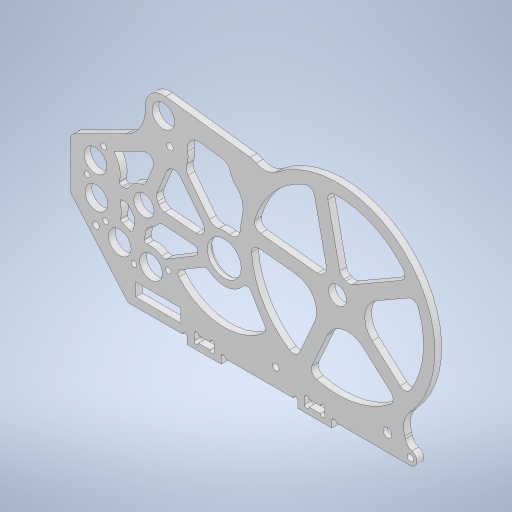
# Autodesk Inventor part: 右フレーム
Saved by Autodesk Inventor 2023.1 (Build 271208000, 208)
## iProperties
Created: 2022-06-19
Part Number: 右フレーム
Material: アルミニウム 2014-T6
Document SubType Name: Modeling
Designer: muzho
Density: 2.78927 g/cm^3
Appearance: サテン
Mass: 58.0664 g
Surface Area: 187.027 cm^2
Volume: 20.8178 cm^3
Author: muzho
Autodesk Inventor part; units mm, degrees
ref_plane "YZ Plane" through (0, 0, 0) normal (1, 0, 0) x (0, 1, 0)
ref_plane "XZ Plane" through (0, 0, 0) normal (0, 1, 0) x (-1, 0, 0)
ref_plane "XY Plane" through (0, 0, 0) normal (0, 0, 1) x (1, 0, 0)
sketch "スケッチ1" plane through (0, 0, 0) normal (0, 0, 1) x (1, 0, 0)
  circle A0 centre (-51.0684, 48.1873) radius 1.3
  circle A1 centre (-58.3027, 33.9162) radius 1.3
  circle A2 centre (-50.1964, 20.1218) radius 1.3
  circle A3 centre (-37.7457, 10.0728) radius 1.3
  circle A4 centre (-22.565, 15.1272) radius 1.3
  circle A5 centre (-33.2954, 34.6933) radius 22.3153 construction
  circle A6 centre (2.1359, 32) radius 30.9835 construction
  circle A7 centre (52, 42.9528) radius 41.9528 construction
  circle A8 centre (2.1208, 32.0012) radius 10.5
  circle A9 centre (-33.2954, 34.6933) radius 6.4335 construction
  circle A10 centre (-54.6856, 41.0518) radius 5.025
  circle A11 centre (-54.2496, 27.019) radius 5.025
  circle A12 centre (-43.9711, 15.0973) radius 5.025
  circle A13 centre (-30.1554, 12.6) radius 5.025
  circle A14 centre (-21.8214, 62.7533) radius 3
  circle A15 centre (-21.8214, 62.7533) radius 8
  line L0 (-21.8214, 62.7533) -> (-51.0684, 48.1873) construction
  line L1 (-33.3165, 55.1292) -> (-46.2281, 48.6988)
  arc A16 (-46.2281, 48.6988) -> (-46.7797, 47.8761) centre (-45.7823, 47.8037) ccw
  arc A17 (-52.9854, 52.0364) -> (-52.4722, 52.2518) centre (-51.0684, 48.1873) ccw construction
  arc A18 (-45.8061, 47.5867) -> (-65.5671, 39.279) centre (-54.6856, 41.0518) ccw construction
  line L2 (-65.7532, 43.7746) -> (-65.4452, 23.4769)
  arc A19 (-63.3575, 39.1831) -> (-63.6558, 28.9529) centre (-58.3027, 33.9162) ccw construction
  arc A20 (-45.2817, 33.4322) -> (-57.345, 16.4375) centre (-54.2496, 27.019) ccw construction
  arc A21 (-54.981, 15.674) -> (-41.5533, 4.3407) centre (-43.9711, 15.0973) ccw construction
  arc A22 (-65.4452, 23.4769) -> (-65.2027, 22.8391) centre (-64.4453, 23.4921) ccw
  line L3 (-65.2027, 22.8391) -> (-40.6377, -5.653)
  arc A23 (-40.6377, -5.653) -> (-39.8804, -6) centre (-39.8804, -5) ccw
  line L4 (-39.8804, -6) -> (84.0728, -6)
  line L5 (-6.7219, 36.0268) -> (-6.7219, -6.1434) construction
  line L6 (-37.0636, -3) -> (111.1776, -3) construction
  circle A24 centre (-10.2219, -3) radius 1
  circle A25 centre (-10.2219, -6) radius 1
  circle A26 centre (-15.2219, -6) radius 1
  line L7 (-11.2219, -3) -> (-11.2219, -6)
  circle A27 centre (-3.2219, -3) radius 1
  line L8 (-2.2219, -3) -> (-2.2219, -6)
  circle A28 centre (-3.2219, -6) radius 1
  circle A29 centre (1.7781, -6) radius 1
  line L9 (-9.2219, -3) -> (-4.2219, -3)
  line L10 (-14.2219, -6) -> (-14.2219, -9)
  line L11 (-14.2219, -9) -> (-7.7219, -9)
  line L12 (0.7781, -9) -> (-7.7219, -9)
  line L13 (0.7781, -6) -> (0.7781, -9)
  circle A30 centre (-33.2954, 34.6933) radius 4.5
  circle A31 centre (-33.2954, 34.6933) radius 7.5
  line L14 (-54.6856, 41.0518) -> (-54.2496, 27.019) construction
  line L15 (-54.4676, 34.0354) -> (-33.2954, 34.6933) construction
  arc A32 (-46.934, 49.3692) -> (-46.3247, 48.2383) centre (-44.0496, 50.1938) ccw
  arc A33 (-44.0483, 38.1537) -> (-46.3247, 48.2383) centre (-54.6856, 41.0518) ccw
  line L16 (-43.0524, 36.8913) -> (-42.313, 36.9143)
  line L17 (-42.8971, 31.8937) -> (-42.1577, 31.9167)
  arc A34 (-44.0483, 38.1537) -> (-43.0524, 36.8913) centre (-43.0835, 37.8908) ccw
  arc A35 (-42.8971, 31.8937) -> (-43.8127, 30.5719) centre (-42.8661, 30.8942) ccw
  arc A36 (-43.5733, 24.2678) -> (-43.8127, 30.5719) centre (-54.2496, 27.019) ccw
  arc A37 (-43.5733, 24.2678) -> (-42.7563, 23.0298) centre (-42.605, 24.0183) ccw
  arc A38 (-39.5768, 21.8123) -> (-42.7563, 23.0298) centre (-43.9711, 15.0973) ccw
  arc A39 (-42.313, 36.9143) -> (-39.8031, 38.4215) centre (-42.4062, 39.9128) ccw
  arc A40 (-39.5591, 30.5682) -> (-42.1577, 31.9167) centre (-42.0645, 28.9181) ccw
  arc A41 (-39.5768, 21.8123) -> (-38.0451, 22.4712) centre (-39.0292, 22.649) ccw
  line L18 (-38.0451, 22.4712) -> (-37.3465, 26.3363)
  line L19 (-43.9711, 15.0973) -> (-30.1554, 12.6) construction
  line L20 (-37.0632, 13.8486) -> (-33.2954, 34.6933) construction
  line L21 (-32.4262, 25.4469) -> (-33.1249, 21.5818)
  arc A42 (-33.1249, 21.5818) -> (-31.9208, 20.4284) centre (-32.1408, 21.4039) ccw
  arc A43 (-25.4982, 19.1354) -> (-31.9208, 20.4284) centre (-30.1554, 12.6) ccw
  arc A44 (-37.3465, 26.3363) -> (-38.2977, 29.1052) centre (-40.2986, 26.8699) ccw
  arc A45 (-30.5659, 27.7076) -> (-32.4262, 25.4469) centre (-29.4741, 24.9133) ccw
  arc A46 (-32.898, 62.0405) -> (-29.1429, 65.9774) centre (-36.4645, 69.2016) ccw
  line L22 (-21.8214, 62.7533) -> (-33.2954, 34.6933) construction
  line L23 (-29.2023, 51.3083) -> (-32.2241, 43.9183)
  line L24 (-23.2251, 52.7152) -> (-27.5961, 42.0259)
  arc A47 (-34.5136, 42.0937) -> (-32.2241, 43.9183) centre (-35.0009, 45.0538) ccw
  arc A48 (-27.5961, 42.0259) -> (-27.241, 39.1198) centre (-24.8193, 40.8904) ccw
  arc A49 (-29.2023, 51.3083) -> (-33.3165, 55.1292) centre (-31.9791, 52.4438) ccw
  circle A50 centre (2.1208, 32.0012) radius 7.5
  circle A51 centre (2.1208, 32.0012) radius 8.5
  arc A52 (-25.4982, 19.1354) -> (-23.3071, 19.05) centre (-24.3375, 20.7641) ccw
  line L25 (-23.3071, 19.05) -> (-10.4064, 26.8046)
  line L26 (-30.1554, 12.6) -> (2.1208, 32.0012) construction
  arc A53 (-26.6272, 38.1263) -> (-24.1874, 36.5081) centre (-23.96, 39.4995) ccw
  arc A54 (-24.5663, 31.5225) -> (-27.2228, 30.2917) centre (-24.7937, 28.5311) ccw
  line L27 (-24.1874, 36.5081) -> (-10.2124, 35.4459)
  line L28 (-24.5663, 31.5225) -> (-11.2852, 30.513)
  line L29 (-33.2954, 34.6933) -> (2.1208, 32.0012) construction
  arc A55 (-10.4064, 26.8046) -> (-11.2852, 30.513) centre (-11.4368, 28.5187) ccw
  circle A56 centre (-54.6856, 41.0518) radius 14 construction
  line L30 (42, 44.1233) -> (42, -23.5713) construction
  circle A57 centre (38.5, -3) radius 1
  circle A58 centre (38.5, -6) radius 1
  circle A59 centre (33.5, -6) radius 1
  line L31 (37.5, -3) -> (37.5, -6)
  line L32 (34.5, -6) -> (34.5, -9)
  line L33 (34.5, -9) -> (42, -9)
  circle A60 centre (45.5, -3) radius 1
  line L34 (46.5, -3) -> (46.5, -6)
  circle A61 centre (45.5, -6) radius 1
  line L35 (49.5, -6) -> (49.5, -9)
  line L36 (49.5, -9) -> (42, -9)
  circle A62 centre (50.5, -6) radius 1
  line L37 (39.5, -3) -> (44.5, -3)
  circle A63 centre (52, 42.9528) radius 4.025
  circle A64 centre (52, 42.9528) radius 8.025
  arc A65 (83.7206, 13.9916) -> (24.9838, 76.3454) centre (52, 42.9528) ccw
  line L38 (52, 42.9528) -> (49.2725, 42.9528) construction
  arc A66 (55.6469, 50.1013) -> (58.5102, 50.1755) centre (57.0102, 52.7736) ccw
  line L39 (58.5102, 50.1755) -> (80.3207, 62.7679)
  arc A67 (80.3207, 62.7679) -> (81.1227, 67.2896) centre (78.8207, 65.3659) ccw
  arc A68 (61.5102, 44.9794) -> (60.0142, 42.5368) centre (63.0102, 42.3813) ccw
  arc A69 (87.6377, 56.0054) -> (83.3207, 57.5717) centre (84.8207, 54.9736) ccw
  line L40 (61.5102, 44.9794) -> (83.3207, 57.5717)
  line L41 (52, 42.9528) -> (85.5729, 62.3361) construction
  line L42 (52, 42.9528) -> (90.7666, 42.9528) construction
  line L43 (47.1425, 51.3763) -> (41.9063, 76.0106)
  arc A70 (46.3283, 48.6302) -> (47.1425, 51.3763) centre (44.2081, 50.7526) ccw
  arc A71 (41.9063, 76.0106) -> (37.8537, 78.1706) centre (38.9719, 75.3868) ccw
  arc A72 (50.5989, 80.8797) -> (47.7752, 77.258) centre (50.7097, 77.8818) ccw
  line L44 (53.0114, 52.6238) -> (47.7752, 77.258)
  arc A73 (53.0114, 52.6238) -> (54.8721, 50.4462) centre (55.9458, 53.2475) ccw
  line L45 (42.4877, 40.936) -> (17.4411, 43.5686)
  arc A74 (44.8478, 39.3131) -> (42.4877, 40.936) centre (42.1741, 37.9525) ccw
  arc A75 (17.4411, 43.5686) -> (14.1344, 40.3818) centre (17.1275, 40.585) ccw
  arc A76 (15.4964, 53.3403) -> (18.0683, 49.5357) centre (18.3818, 52.5193) ccw
  line L46 (43.1149, 46.9032) -> (18.0683, 49.5357)
  arc A77 (43.1149, 46.9032) -> (45.7609, 48) centre (43.4285, 49.8867) ccw
  line L47 (50.9786, 33.2829) -> (40.7351, 10.2756)
  arc A78 (53.2514, 35.026) -> (50.9786, 33.2829) centre (53.7192, 32.0627) ccw
  arc A79 (40.7351, 10.2756) -> (42.7441, 6.146) centre (43.4757, 9.0554) ccw
  arc A80 (30.8406, 11.4457) -> (35.2538, 12.716) centre (32.5132, 13.9362) ccw
  line L48 (45.4973, 35.7233) -> (35.2538, 12.716)
  arc A81 (45.4973, 35.7233) -> (45.2719, 38.5787) centre (42.7567, 36.9435) ccw
  line L49 (60.881, 38.9932) -> (79.5968, 22.1414)
  arc A82 (59.9256, 41.6934) -> (60.881, 38.9932) centre (62.8884, 41.2226) ccw
  arc A83 (79.5968, 22.1414) -> (84.1451, 22.776) centre (81.6042, 24.3708) ccw
  arc A84 (75.4264, 13.0928) -> (75.582, 17.6825) centre (73.5746, 15.4531) ccw
  line L50 (56.8662, 34.5343) -> (75.582, 17.6825)
  arc A85 (56.8662, 34.5343) -> (54.0809, 35.2023) centre (54.8588, 32.3049) ccw
  circle A86 centre (52, 42.9528) radius 37.9528
  circle A87 centre (-33.5773, 1) radius 1.5 construction
  circle A88 centre (-33.5773, 1) radius 3 construction
  line L51 (-39.8804, -5) -> (-33.5773, 1) construction
  circle A89 centre (24.8719, 2) radius 1.5
  circle A90 centre (24.8719, 2) radius 3
  line L52 (24.8719, 10.9511) -> (24.8719, -6.9511) construction
  circle A91 centre (84.0728, -3) radius 1.5
  circle A92 centre (84.0728, -3) radius 3
  arc A93 (-17.1874, 53.5456) -> (-23.2251, 52.7152) centre (-19.9659, 51.3824) ccw
  line L53 (-21.8214, 62.7533) -> (2.1208, 32.0012) construction
  line L54 (-17.1874, 53.5456) -> (-7.3085, 40.8568)
  arc A94 (-10.2124, 35.4459) -> (-7.3085, 40.8568) centre (-9.9579, 38.794) ccw
  arc A95 (10.184, 52.7694) -> (9.1488, 45.9046) centre (52, 42.9528) ccw
  arc A96 (-4.6743, 23.9963) -> (10.5141, 25.6922) centre (2.1208, 32.0012) ccw
  arc A97 (-4.6743, 23.9963) -> (-6.999, 24.1858) centre (-5.9686, 22.4716) ccw
  line L55 (-6.999, 24.1858) -> (-17.3917, 17.9387)
  arc A98 (-17.3917, 17.9387) -> (-17.8825, 14.9261) centre (-16.3614, 16.2245) ccw
  arc A99 (-20.5941, 11.3055) -> (-18.526, 16.6024) centre (-22.565, 15.1272) ccw construction
  arc A100 (-17.8825, 14.9261) -> (19.7697, 12.5022) centre (2.1208, 32.0012) ccw
  arc A101 (13.8269, 25.5208) -> (10.5141, 25.6922) centre (12.1128, 24.4905) ccw
  line L56 (13.8269, 25.5208) -> (20.1417, 15.0154)
  arc A102 (19.7697, 12.5022) -> (20.1417, 15.0154) centre (18.4276, 13.985) ccw
  arc A103 (16.2511, 75.4723) -> (24.9838, 76.3454) centre (19.952, 82.5648) ccw
  circle A104 centre (12.5499, 68.38) radius 4
  circle A105 centre (12.5499, 68.38) radius 8
  circle A106 centre (74.0428, 1.5165) radius 2
  arc A107 (76.7818, -6) -> (71.3037, -6) centre (74.0428, 1.5165) ccw
  arc A108 (83.7206, 13.9916) -> (81.6262, 4.0643) centre (91.1055, 7.2491) ccw
  arc A109 (81.8996, 3.0231) -> (84.8251, -0.0958) centre (85.8281, 3.7764) ccw
  arc A110 (-64.0909, 46.5055) -> (-65.7532, 43.7746) centre (-62.7535, 43.8201) ccw
  line L57 (-64.0909, 46.5055) -> (-32.898, 62.0405)
  circle A111 centre (2.1208, 32.0012) radius 11.5 construction
  circle A112 centre (74.0428, 1.5165) radius 3
  circle A113 centre (74.0428, 1.5165) radius 4
  circle A114 centre (12.5499, 68.38) radius 2
  circle A115 centre (-21.8214, 62.7533) radius 1.5
  circle A116 centre (-54.4309, 16.4709) radius 1.5
  circle A117 centre (-54.4309, 16.4709) radius 3
  arc A118 (-58.2926, 17.5135) -> (-53.5618, 12.5665) centre (-54.4309, 16.4709) ccw construction
  line L58 (-54.2496, 27.019) -> (-43.9711, 15.0973)
  line L59 (-54.4309, 16.4709) -> (-49.1103, 21.0581)
  arc A119 (68.9958, 49.3012) -> (67.3045, 33.2095) centre (73.9958, 40.6409) ccw
  arc A120 (63.2897, 28.7506) -> (47.4629, 25.3865) centre (56.5984, 21.3192) ccw
  arc A121 (41.9816, 27.827) -> (33.8915, 41.8396) centre (32.8462, 31.8943) ccw
  circle A122 centre (-24.7192, 72.9643) radius 4 construction
  arc A123 (-27.2542, 68.6256) -> (-20.283, 70.6039) centre (-24.7192, 72.9643) ccw
  arc A124 (-29.0291, 66.2245) -> (-17.5115, 69.493) centre (-24.7192, 72.9643) ccw construction
  arc A125 (-17.5115, 69.493) -> (-29.0291, 66.2245) centre (-24.7192, 72.9643) ccw
  arc A126 (-40.9817, 58.0146) -> (-32.7016, 72.4347) centre (-47.6687, 71.4416) ccw
  line L60 (-23.7425, 80.9044) -> (13.5266, 76.3201)
  arc A127 (4.7383, 66.6541) -> (1.3208, 69.7612) centre (0.8325, 65.7911) ccw
  line L61 (1.3208, 69.7612) -> (-8.6288, 70.9851)
  arc A128 (-8.6288, 70.9851) -> (-14.0785, 64.7651) centre (-9.2392, 66.0225) ccw
  arc A129 (10.184, 52.7694) -> (7.1716, 62.4577) centre (0.4487, 55.0548) ccw
  arc A130 (4.3203, 42.2682) -> (9.1488, 45.9046) centre (5.1582, 46.1794) ccw
  arc A131 (-14.409, 59.7438) -> (-13.8591, 55.7818) centre (-10.7028, 58.2391) ccw
  line L62 (-13.8591, 55.7818) -> (-4.4104, 43.6456)
  arc A132 (-4.4104, 43.6456) -> (-0.3231, 42.2128) centre (-1.2542, 46.1029) ccw
  line L63 (-24.7192, 72.9643) -> (2.1208, 32.0012) construction
  arc A133 (-20.283, 70.6039) -> (-27.2542, 68.6256) centre (-24.7192, 72.9643) ccw
  line L64 (-16.9824, 3.575) -> (-16.9824, -2.2414)
  line L65 (-36.9824, 3.575) -> (-16.9824, 3.575)
  line L66 (-16.9824, -2.2414) -> (-36.9824, -2.2414)
  line L67 (-36.9824, -2.2414) -> (-36.9824, 3.575)
  point P0 (0, 0)
  point P1 (0, 0)
  point P2 (29.8767, 73.7907)
  point P3 (16.7177, 56.9376)
  point P4 (46.0783, 56.3832)
  point P5 (-16.2219, -6)
  point P6 (0.7781, -6)
  point P7 (2.7781, -6)
  point P8 (32.5, -6)
  point P9 (51.5, -6)
  point P10 (-43.2615, 31.8127)
  point P11 (-43.4211, 36.9495)
  point P12 (-46.5149, 48.4843)
  point P13 (0.7781, -6)
  point P14 (-4.2219, -6)
  point P15 (-9.2219, -6)
  point P16 (44.5, -6)
  point P17 (39.5, -6)
  point P18 (81.3373, -1.7682)
  point P19 (54.8721, 50.4462)
  point P20 (50.5989, 80.8797)
  point P21 (15.4964, 53.3403)
  point P22 (14.1344, 40.3818)
  point P23 (44.8478, 39.3131)
  point P24 (45.2719, 38.5787)
  point P25 (30.8406, 11.4457)
  point P26 (42.7441, 6.146)
  point P27 (53.2514, 35.026)
  point P28 (54.0809, 35.2023)
  point P29 (75.4264, 13.0928)
  point P30 (84.1451, 22.776)
  point P31 (59.9256, 41.6934)
  point P32 (64.0505, 41.6862)
  point P33 (54.5192, 31.1007)
  point P34 (41.5064, 36.8943)
  point P35 (45.7609, 48)
  point P36 (46.3283, 48.6302)
  point P37 (-24.4592, 70.3059)
  point P38 (15.8273, 75.6778)
  point P39 (-20.533, 54.8577)
  point P40 (-7.0312, 37.1481)
  dimension "d7" = 16
  dimension "d19" = 3
  dimension "d21" = 2
  dimension "d22" = 2
  dimension "d59" = 2
  dimension "d60" = 2
  dimension "d2" = 10.05
  dimension "d3" = 10.05
  dimension "d4" = 10.05
  dimension "d5" = 10.05
  dimension "d6" = 6
  dimension "d8" = 1
  dimension "d9" = 3
  dimension "d10" = 6
  dimension "d11" = 6
  dimension "d12" = 6
  dimension "d13" = 1
  dimension "d14" = 6
  dimension "d15" = 1
  dimension "d16" = 6
  dimension "d17" = 35.4313
  dimension "d18" = 8.8578
  dimension "d20" = 2
  dimension "d23" = 5
  dimension "d24" = 3.5
  dimension "d25" = 3
  dimension "d26" = 9
  dimension "d27" = 3
  dimension "d28" = 3
  dimension "d29" = 5
  dimension "d30" = 2.5
  dimension "d31" = 1
  dimension "d32" = 1
  dimension "d33" = 3
  dimension "d34" = 1
  dimension "d35" = 3
  dimension "d36" = 3
  dimension "d37" = 1
  dimension "d38" = 1
  dimension "d39" = 3
  dimension "d40" = 5
  dimension "d41" = 2.5
  dimension "d42" = 3
  dimension "d43" = 3
  dimension "d44" = 8
  dimension "d45" = 3
  dimension "d46" = 3
  dimension "d47" = 5
  dimension "d48" = 2.5
  dimension "d49" = 3
  dimension "d50" = 15
  dimension "d51" = 2
  dimension "d52" = 2
  dimension "d53" = 3
  dimension "d54" = 3
  dimension "d55" = 5
  dimension "d56" = 2.5
  dimension "d57" = 2
  dimension "d58" = 2
  dimension "d61" = 3.5
  dimension "d62" = 5
  dimension "d63" = 3
  dimension "d64" = 8.05
  dimension "d65" = 4
  dimension "d66" = 1
  dimension "d67" = 3
  dimension "d68" = 3
  dimension "d69" = 3
  dimension "d70" = 30
  dimension "d71" = 6
  constraints: 194 point on circle, 132 end point, 123 centre point, 85 tangent, 25 coincident, 17 parallel, 15 concentric, 14 symmetric about line, 12 vertical, 6 horizontal, 5 point on line, 4 midpoint, 3 perpendicular, 2 vertical alignment, 1 equal length, 1 equal radius, 218 other
  measures "d2" diameter of A10
  measures "d3" diameter of A11
  measures "d4" diameter of A12
  measures "d5" diameter of A13
  measures "d6" diameter of A14
  measures "d8" radius of A16
  measures "d9" radial gap between concentric circles of A0 A17
  measures "d10" radial gap between concentric circles of A10 A18
  measures "d11" radial gap between concentric circles of A1 A19
  measures "d12" radial gap between concentric circles of A20 A11
  measures "d13" radius of A22
  measures "d14" radial gap between concentric circles of A21 A12
  measures "d15" radius of A23
  measures "d17" horizontal distance of point (2.136, 32) A5.centre
  measures "d18" distance from line of point (2.136, 32) L5
  measures "d20" diameter of A24
  measures "d23" distance of point (-10.222, -6) point (-15.222, -6)
  measures "d24" distance from line of L5 A24.centre
  measures "d25" distance of L10.start L10.end
  measures "d26" diameter of A30
  measures "d28" radius of A32
  measures "d29" distance between parallel lines of L17 L16
  measures "d30" distance between parallel lines of L17 L15
  measures "d31" radius of A34
  measures "d32" radius of A35
  measures "d33" radial gap between concentric circles of A12 A38
  measures "d34" radius of A37
  measures "d35" radius of A39
  measures "d36" radius of A40
  measures "d37" radius of A41
  measures "d38" radius of A42
  measures "d39" radial gap between concentric circles of A13 A43
  measures "d40" distance between parallel lines of L21 L18
  measures "d41" distance between parallel lines of L20 L21
  measures "d42" radius of A45
  measures "d43" radius of A44
  measures "d44" radius of A46
  measures "d45" radius of A47
  measures "d46" radius of A48
  measures "d47" distance between parallel lines of L24 L23
  measures "d48" distance between parallel lines of L24 L22
  measures "d49" radius of A49
  measures "d50" diameter of A50
  measures "d51" radius of A52
  measures "d52" distance between parallel lines of L26 L25
  measures "d53" radius of A53
  measures "d54" radius of A54
  measures "d55" distance between parallel lines of L28 L27
  measures "d56" distance between parallel lines of L28 L29
  measures "d57" radius of A55
  measures "d58" diameter of A57
  measures "d61" distance from line of L30 A57.centre
  measures "d62" distance of point (38.5, -6) point (33.5, -6)
  measures "d63" distance of L32.start L32.end
  measures "d64" diameter of A63
  measures "d65" radial gap between concentric circles of A63 A64
  measures "d67" radius of A66
  measures "d68" radius of A67
  measures "d69" radius of A68
  measures "d70" angle of L42 L41
  measures "d71" distance between parallel lines of L39 L40
extrude "押し出し1" add sketch "スケッチ1" against normal blind 3 contours A8 | A8 A130 A95 A129 A105 A103 A65 A108 A107 L4 A62 L34 A60 L37 A57 L31 A59 A29 L8 A27 L9 A24 L7 A26 A23 L3 A22 L2 A110 L57 A46 A15 A93 L24 A48 A31 A47 L23 A49 L1 A16 A32 A33 A34 L16 A39 A40 L17 A35 A36 A37 A38 A41 L18 A44 A45 L21 A42 A43 A52 L25 A55 L28 A54 A53 L27 A94 A97 L55 A98 A100 A102 L56 A101 | A8 A94 L54 A93 A15 A131 L62 A132 | A105 | A15 A123 | A127 L61 A128 A15 A125 L60 A105 | A31 | A46 L57 A126 A125 A15 | A125 A15 A133 | A107 L4 | A109 A92 A107 | A92 | A92 L4 A107 | L35 L36 L33 L32 L4 A58 A61 | L4 A25 A28 L13 L12 L11 L10 | A14 | A64 | A64 A66 L39 A67 A86 A69 L40 A68 | A68 L40 A119 L49 A82 A64 | A64 A70 L43 A71 A86 A72 L44 A73 | A82 L49 A83 A86 A84 L50 A85 A64 | A85 L50 A120 L47 A78 A64 | A64 A74 L45 A75 A86 A76 L46 A77 | A78 L47 A79 A86 A80 L48 A81 A64 | A64 A81 L48 A121 L45 A74 | A90 | A104 | A114 | A117 picked at (-26.405, 66.4688)
extrude "押し出し2" add sketch "スケッチ1" against normal blind 1.8 contours A51 | A112 | A113
fillet "フィレット1" radius 1 1 edges at (70.0428, 1.5165, -1.8)
sketch "スケッチ2" plane through (0, 0, -3) normal (0, 0, -1) x (-1, 0, 0)
  arc A0 (-50.5989, 80.8797) -> (-81.1227, 67.2896) centre (-52, 42.9528) ccw projected
  arc A1 (-47.7752, 77.258) -> (-50.5989, 80.8797) centre (-50.7097, 77.8818) ccw projected
  line L0 (-47.7752, 77.258) -> (-53.0114, 52.6238) projected
  arc A2 (-54.8721, 50.4462) -> (-53.0114, 52.6238) centre (-55.9458, 53.2475) ccw projected
  arc A3 (-54.8721, 50.4462) -> (-55.6469, 50.1013) centre (-52, 42.9528) ccw projected
  arc A4 (-58.5102, 50.1755) -> (-55.6469, 50.1013) centre (-57.0102, 52.7736) ccw projected
  line L1 (-58.5102, 50.1755) -> (-80.3207, 62.7679) projected
  arc A5 (-81.1227, 67.2896) -> (-80.3207, 62.7679) centre (-78.8207, 65.3659) ccw projected
  circle A6 centre (-52, 42.9528) radius 4.025 projected
  line L2 (9.2219, -6) -> (4.2219, -6) projected
  line L3 (-39.5, -6) -> (-44.5, -6) projected
  circle A7 centre (-84.0728, -3) radius 1.5 projected
  arc A8 (-13.5266, 76.3201) -> (-16.2511, 75.4723) centre (-12.5499, 68.38) ccw projected
  arc A9 (-84.8251, -0.0958) -> (-81.8996, 3.0231) centre (-85.8281, 3.7764) ccw projected
  arc A10 (-84.8251, -0.0958) -> (-84.0728, -6) centre (-84.0728, -3) ccw projected
  line L4 (-84.0728, -6) -> (-51.5, -6) projected
  arc A11 (16.2219, -6) -> (14.2219, -6) centre (15.2219, -6) ccw projected
  line L5 (16.2219, -6) -> (39.8804, -6) projected
  arc A12 (-15.4964, 53.3403) -> (-37.8537, 78.1706) centre (-52, 42.9528) ccw projected
  arc A13 (-18.0683, 49.5357) -> (-15.4964, 53.3403) centre (-18.3818, 52.5193) ccw projected
  line L6 (-18.0683, 49.5357) -> (-43.1149, 46.9032) projected
  arc A14 (-45.7609, 48) -> (-43.1149, 46.9032) centre (-43.4285, 49.8867) ccw projected
  arc A15 (-45.7609, 48) -> (-46.3283, 48.6302) centre (-52, 42.9528) ccw projected
  arc A16 (-47.1425, 51.3763) -> (-46.3283, 48.6302) centre (-44.2081, 50.7526) ccw projected
  line L7 (-47.1425, 51.3763) -> (-41.9063, 76.0106) projected
  arc A17 (-37.8537, 78.1706) -> (-41.9063, 76.0106) centre (-38.9719, 75.3868) ccw projected
  arc A18 (-30.8406, 11.4457) -> (-14.1344, 40.3818) centre (-52, 42.9528) ccw projected
  arc A19 (-35.2538, 12.716) -> (-30.8406, 11.4457) centre (-32.5132, 13.9362) ccw projected
  line L8 (-35.2538, 12.716) -> (-41.9816, 27.827) projected
  arc A20 (-33.8915, 41.8396) -> (-41.9816, 27.827) centre (-32.8462, 31.8943) ccw projected
  line L9 (-33.8915, 41.8396) -> (-17.4411, 43.5686) projected
  arc A21 (-14.1344, 40.3818) -> (-17.4411, 43.5686) centre (-17.1275, 40.585) ccw projected
  arc A22 (-75.4264, 13.0928) -> (-42.7441, 6.146) centre (-52, 42.9528) ccw projected
  arc A23 (-75.582, 17.6825) -> (-75.4264, 13.0928) centre (-73.5746, 15.4531) ccw projected
  line L10 (-75.582, 17.6825) -> (-63.2897, 28.7506) projected
  arc A24 (-47.4629, 25.3865) -> (-63.2897, 28.7506) centre (-56.5984, 21.3192) ccw projected
  line L11 (-47.4629, 25.3865) -> (-40.7351, 10.2756) projected
  arc A25 (-42.7441, 6.146) -> (-40.7351, 10.2756) centre (-43.4757, 9.0554) ccw projected
  arc A26 (-84.1451, 22.776) -> (-79.5968, 22.1414) centre (-81.6042, 24.3708) ccw projected
  arc A27 (-87.6377, 56.0054) -> (-84.1451, 22.776) centre (-52, 42.9528) ccw projected
  arc A28 (-83.3207, 57.5717) -> (-87.6377, 56.0054) centre (-84.8207, 54.9736) ccw projected
  line L12 (-83.3207, 57.5717) -> (-68.9958, 49.3012) projected
  arc A29 (-67.3045, 33.2095) -> (-68.9958, 49.3012) centre (-73.9958, 40.6409) ccw projected
  line L13 (-67.3045, 33.2095) -> (-79.5968, 22.1414) projected
  arc A30 (-81.6262, 4.0643) -> (-81.8996, 3.0231) centre (-74.0428, 1.5165) ccw projected
  line L14 (-46.5, -6) -> (-46.5, -3) projected
  arc A31 (-44.5, -3) -> (-46.5, -3) centre (-45.5, -3) ccw projected
  line L15 (-44.5, -3) -> (-39.5, -3) projected
  arc A32 (-37.5, -3) -> (-39.5, -3) centre (-38.5, -3) ccw projected
  line L16 (-37.5, -3) -> (-37.5, -6) projected
  line L17 (2.2219, -6) -> (2.2219, -3) projected
  arc A33 (4.2219, -3) -> (2.2219, -3) centre (3.2219, -3) ccw projected
  line L18 (4.2219, -3) -> (9.2219, -3) projected
  arc A34 (11.2219, -3) -> (9.2219, -3) centre (10.2219, -3) ccw projected
  line L19 (11.2219, -3) -> (11.2219, -6) projected
  arc A35 (0.3231, 42.2128) -> (-4.3203, 42.2682) centre (-2.1208, 32.0012) ccw projected
  arc A36 (-49.5, -6) -> (-51.5, -6) centre (-50.5, -6) ccw projected
  arc A37 (-32.5, -6) -> (-34.5, -6) centre (-33.5, -6) ccw projected
  arc A38 (-0.7781, -6) -> (-2.7781, -6) centre (-1.7781, -6) ccw projected
  line L20 (-32.5, -6) -> (-2.7781, -6) projected
  line L21 (23.7425, 80.9044) -> (-13.5266, 76.3201) projected
  arc A39 (-24.9838, 76.3454) -> (-16.2511, 75.4723) centre (-19.952, 82.5648) ccw projected
  arc A40 (-24.9838, 76.3454) -> (-83.7206, 13.9916) centre (-52, 42.9528) ccw projected
  arc A41 (-81.6262, 4.0643) -> (-83.7206, 13.9916) centre (-91.1055, 7.2491) ccw projected
  line L22 (-49.5, -6) -> (-49.5, -9) projected
  line L23 (-49.5, -9) -> (-34.5, -9) projected
  line L24 (-34.5, -9) -> (-34.5, -6) projected
  line L25 (-0.7781, -6) -> (-0.7781, -9) projected
  line L26 (-0.7781, -9) -> (14.2219, -9) projected
  line L27 (14.2219, -9) -> (14.2219, -6) projected
  arc A42 (39.8804, -6) -> (40.6377, -5.653) centre (39.8804, -5) ccw projected
  line L28 (40.6377, -5.653) -> (65.2027, 22.8391) projected
  arc A43 (65.2027, 22.8391) -> (65.4452, 23.4769) centre (64.4453, 23.4921) ccw projected
  line L29 (65.4452, 23.4769) -> (65.7532, 43.7746) projected
  arc A44 (65.7532, 43.7746) -> (64.0909, 46.5055) centre (62.7535, 43.8201) ccw projected
  line L30 (64.0909, 46.5055) -> (40.9817, 58.0146) projected
  arc A45 (32.7016, 72.4347) -> (40.9817, 58.0146) centre (47.6687, 71.4416) ccw projected
  arc A46 (32.7016, 72.4347) -> (23.7425, 80.9044) centre (24.7192, 72.9643) ccw projected
  arc A47 (9.2219, -6) -> (11.2219, -6) centre (10.2219, -6) ccw projected
  arc A48 (2.2219, -6) -> (4.2219, -6) centre (3.2219, -6) ccw projected
  arc A49 (-39.5, -6) -> (-37.5, -6) centre (-38.5, -6) ccw projected
  arc A50 (-46.5, -6) -> (-44.5, -6) centre (-45.5, -6) ccw projected
  arc A51 (14.0785, 64.7651) -> (14.409, 59.7438) centre (21.8214, 62.7533) ccw projected
  arc A52 (-10.5141, 25.6922) -> (-13.8269, 25.5208) centre (-12.1128, 24.4905) ccw projected
  arc A53 (-10.5141, 25.6922) -> (4.6743, 23.9963) centre (-2.1208, 32.0012) ccw projected
  arc A54 (6.999, 24.1858) -> (4.6743, 23.9963) centre (5.9686, 22.4716) ccw projected
  line L31 (6.999, 24.1858) -> (17.3917, 17.9387) projected
  arc A55 (17.8825, 14.9261) -> (17.3917, 17.9387) centre (16.3614, 16.2245) ccw projected
  arc A56 (-19.7697, 12.5022) -> (17.8825, 14.9261) centre (-2.1208, 32.0012) ccw projected
  arc A57 (-20.1417, 15.0154) -> (-19.7697, 12.5022) centre (-18.4276, 13.985) ccw projected
  line L32 (-20.1417, 15.0154) -> (-13.8269, 25.5208) projected
  arc A58 (-7.1716, 62.4577) -> (-4.7383, 66.6541) centre (-12.5499, 68.38) ccw projected
  arc A59 (-1.3208, 69.7612) -> (-4.7383, 66.6541) centre (-0.8325, 65.7911) ccw projected
  line L33 (-1.3208, 69.7612) -> (8.6288, 70.9851) projected
  arc A60 (14.0785, 64.7651) -> (8.6288, 70.9851) centre (9.2392, 66.0225) ccw projected
  arc A61 (13.8591, 55.7818) -> (14.409, 59.7438) centre (10.7028, 58.2391) ccw projected
  line L34 (13.8591, 55.7818) -> (4.4104, 43.6456) projected
  arc A62 (0.3231, 42.2128) -> (4.4104, 43.6456) centre (1.2542, 46.1029) ccw projected
  arc A63 (-9.1488, 45.9046) -> (-4.3203, 42.2682) centre (-5.1582, 46.1794) ccw projected
  arc A64 (-9.1488, 45.9046) -> (-10.184, 52.7694) centre (-52, 42.9528) ccw projected
  arc A65 (-7.1716, 62.4577) -> (-10.184, 52.7694) centre (-0.4487, 55.0548) ccw projected
  point P0 (0, 0)
sketch "スケッチ3" plane through (0, 0, -3) normal (0, 0, -1) x (-1, 0, 0)
  arc A0 (-19.7697, 12.5022) -> (17.8825, 14.9261) centre (-2.1208, 32.0012) ccw projected
  line L0 (-32.5, -6) -> (-2.7781, -6) projected
  arc A1 (-19.022, 0.6667) -> (-18.8952, 2.5273) centre (-24.8719, 2) ccw
  arc A2 (-14.6263, 5.5039) -> (-18.8952, 2.5273) centre (-15.9068, 2.7909) ccw
  arc A3 (-14.6263, 5.5039) -> (-4.6904, 2.814) centre (-2.1208, 32.0012) ccw
  arc A4 (-19.022, 0.6667) -> (-16.097, -3) centre (-16.097, 0) ccw
  line L1 (-16.097, -3) -> (-4.7781, -3)
  arc A5 (-3.7781, 1.8179) -> (-4.6904, 2.814) centre (-4.7781, 1.8179) ccw
  arc A6 (-4.7781, -3) -> (-3.7781, -2) centre (-4.7781, -2) ccw
  line L2 (-3.7781, 1.8179) -> (-3.7781, -2)
  arc A7 (-0.7781, -6) -> (-2.7781, -6) centre (-1.7781, -6) ccw projected
  arc A8 (0.3142, -2.5909) -> (-5.5639, -4.7087) centre (-1.7781, -6) ccw construction
  arc A9 (-75.4264, 13.0928) -> (-42.7441, 6.146) centre (-52, 42.9528) ccw projected
  circle A10 centre (-74.0428, 1.5165) radius 4 projected
  line L3 (-84.0728, -6) -> (-51.5, -6) projected
  arc A11 (-49.5, -6) -> (-51.5, -6) centre (-50.5, -6) ccw projected
  arc A12 (-60.686, 2.9317) -> (-61.3223, -3) centre (-61.3223, 0) ccw
  arc A13 (-60.686, 2.9317) -> (-52, 2) centre (-52, 42.9528) ccw
  line L4 (-61.3223, -3) -> (-52, -3)
  arc A14 (-52, -3) -> (-52, 2) centre (-52, -0.5) ccw
  arc A15 (-24.9838, 76.3454) -> (-16.2511, 75.4723) centre (-19.952, 82.5648) ccw projected
  arc A16 (-7.1716, 62.4577) -> (-4.7383, 66.6541) centre (-12.5499, 68.38) ccw projected
  arc A17 (-15.4964, 53.3403) -> (-37.8537, 78.1706) centre (-52, 42.9528) ccw projected
  arc A18 (-7.1716, 62.4577) -> (-10.184, 52.7694) centre (-0.4487, 55.0548) ccw projected
  arc A19 (-13.5266, 76.3201) -> (-16.2511, 75.4723) centre (-12.5499, 68.38) ccw projected
  line L5 (23.7425, 80.9044) -> (-13.5266, 76.3201) projected
  arc A20 (-17.3024, 71.8886) -> (-14.863, 72.8127) centre (-19.952, 82.5648) ccw
  arc A21 (-7.6184, 69.2047) -> (-14.863, 72.8127) centre (-12.5499, 68.38) ccw
  arc A22 (-9.1884, 64.6785) -> (-7.6184, 69.2047) centre (-12.5499, 68.38) ccw
  arc A23 (-9.1884, 64.6785) -> (-11.0915, 62.52) centre (-0.4487, 55.0548) ccw
  arc A24 (-16.1722, 62.7896) -> (-18.9974, 67.2007) centre (-52, 42.9528) ccw
  arc A25 (-16.1722, 62.7896) -> (-11.0915, 62.52) centre (-13.5476, 64.2427) ccw
  arc A26 (-17.3024, 71.8886) -> (-18.9974, 67.2007) centre (-16.5798, 68.977) ccw
  arc A27 (-7.6184, 69.2047) -> (-7.6184, 69.2047) centre (-9.6958, 68.8573) ccw
  circle A28 centre (-24.8719, 2) radius 1.5 projected
  point P0 (0, 0)
  point P1 (-7.6184, 69.2047)
  dimension "d161" = 3
  dimension "d163" = 3
  dimension "d164" = 3
  dimension "d165" = 1
  dimension "d166" = 1
  dimension "d167" = 3
  dimension "d168" = 3
  dimension "d169" = 3
  dimension "d172" = 3
  dimension "d173" = 3
  dimension "d175" = 2.5
  dimension "d176" = 3
  dimension "d177" = 3
  dimension "d178" = 3
  dimension "d179" = 3
  dimension "d180" = 3
  dimension "d183" = 4.5
  constraints: 36 point on circle, 18 centre point, 18 tangent, 6 end point, 4 concentric, 2 horizontal, 1 perpendicular, 2 other
  measures "d161" radius of A2
  measures "d163" radial gap between concentric circles of A3 A0
  measures "d164" radius of A4
  measures "d165" radius of A5
  measures "d166" radius of A6
  measures "d167" radial gap between concentric circles of A7 A8
  measures "d168" distance between parallel lines of L0 L1
  measures "d169" radius of A12
  measures "d172" radial gap between concentric circles of A13 A9
  measures "d173" distance between parallel lines of L3 L4
  measures "d175" radius of A14
  measures "d176" radial gap between concentric circles of A20 A15
  measures "d177" radial gap between concentric circles of A17 A24
  measures "d178" radial gap between concentric circles of A18 A23
  measures "d179" radius of A25
  measures "d180" radius of A26
  measures "d183" radial gap between concentric circles of A28 A1
extrude "押し出し3" cut sketch "スケッチ3" against normal blind 1.2 contours A1 A2 A3 A5 L2 A6 L1 A4 | A13 A14 L4 A12 | A27 | A20 A21 A22 A23 A25 A24 A26
equation "\"d18\" = 0.25 * d17"
equation "\"d30\" = 0.5 * d29"
equation "\"d41\" = 0.5 * d40"
equation "\"d48\" = 0.5 * d47"
equation "\"d56\" = 0.5 * d55"
